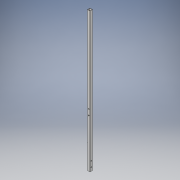
# Autodesk Inventor part: suporte sensores 1m
Saved by Autodesk Inventor 2019.4 (Build 234330000, 330)
## iProperties
Created: 2020-08-25
Part Number: suporte sensores 1m
Material: Alumínio 6061
Document SubType Name: Modeling
Designer: Lattes
Density: 2.7 g/cm^3
Appearance: Alumínio - Polido
Author: Lattes
Autodesk Inventor part; units mm, degrees
ref_plane "YZ Plane" through (0, 0, 0) normal (1, 0, 0) x (0, 1, 0)
ref_plane "XZ Plane" through (0, 0, 0) normal (0, 1, 0) x (-1, 0, 0)
ref_plane "XY Plane" through (0, 0, 0) normal (0, 0, 1) x (1, 0, 0)
sketch "Esboço1" plane through (0, 0, 0) normal (0, 1, 0) x (-1, 0, 0)
  line L0 (0, 0) -> (19.05, 0)
  line L1 (19.05, 0) -> (19.05, -19.05)
  line L2 (19.05, -19.05) -> (0, -19.05)
  line L3 (0, -19.05) -> (0, 0)
  line L4 (17.55, -17.55) -> (17.55, -1.5)
  line L5 (1.5, -1.5) -> (17.55, -1.5)
  line L6 (17.55, -17.55) -> (1.5, -17.55)
  line L7 (1.5, -1.5) -> (1.5, -17.55)
  dimension "d1" = 19.05
  dimension "d2" = 19.05
  dimension "d3" = 19.05
  constraints: 16 end point, 2 perpendicular, 1 horizontal
  measures "d1" distance of L0.start L0.end
  measures "d2" distance of L0.end L1.end
  measures "d3" distance of L1.end L2.end
extrude "Extrusão1" add sketch "Esboço1" along normal blind 1000
sketch "Esboço2" plane through (-19.05, 0, -19.05) normal (0, 0, -1) x (-1, 0, 0)
  point P0 (-19.05, 0)
sketch "Esboço3" plane through (0, 0, 0) normal (0, 0, 1) x (1, 0, 0)
  line L0 (-19.05, 0) -> (0, 0) projected
  line L1 (0, 0) -> (-19.05, 0)
  line L2 (-9.525, 0) -> (-9.525, 480)
  circle A0 centre (-9.525, 479.5) radius 3.5
  circle A1 centre (-9.525, 520.5) radius 3.5
  dimension "d15" = 480
  dimension "d56" = 7
  dimension "d57" = 7
  constraints: 4 end point, 2 centre point, 1 collinear, 1 midpoint, 1 vertical
  measures "d15" distance of L2.start L2.end
  measures "d56" diameter of A0
  measures "d57" diameter of A1
extrude "Extrusão2" cut sketch "Esboço3" against normal blind 20
sketch "Esboço6" plane through (0, 1000, 0) normal (0, 1, 0) x (1, 0, 0)
  line L0 (-19.05, 19.05) -> (0, 19.05) projected
  line L1 (0, 0) -> (-19.05, 0) projected
  line L2 (0, 19.05) -> (-19.05, 19.05)
  line L3 (-19.05, 19.05) -> (-19.05, 0)
  line L4 (-19.05, 0) -> (0, 0)
  line L5 (0, 0) -> (0, 19.05)
  line L6 (-17.55, 1.5) -> (-1.5, 1.5) projected
  line L7 (-17.55, 1.5) -> (-1.5, 1.5)
  line L8 (-1.5, 1.5) -> (-1.5, 17.55)
  line L9 (-1.5, 17.55) -> (-17.55, 17.55)
  line L10 (-17.55, 17.55) -> (-17.55, 1.5)
  constraints: 16 end point, 4 parallel, 2 horizontal, 2 perpendicular
extrude "Extrusão5" add sketch "Esboço6" along normal blind 150
chamfer "Chanfro1" distance 0.5 angle 45 4 edges at (0, 575, 0) (-17.55, 575, -1.5) (-19.05, 575, -19.05) (0, 575, -19.05)
chamfer "Chanfro2" distance 0.5 angle 45 1 edges at (-19.05, 575, 0)
sketch "Esboço7" plane through (-0.5, 0, 0) normal (0, 0, 1) x (1, 0, 0)
  point P0 (0.5, 0)
sketch "Esboço8" plane through (-19.05, 0, -18.55) normal (-1, 0, 0) x (0, 0, 1)
  line L0 (18.55, 1150) -> (16.55, 550.0033)
  line L1 (16.55, 0) -> (16.55, 1150) projected
  line L2 (16.55, 550.0033) -> (16.55, 150.0033)
  line L3 (16.55, 150.0033) -> (1, 150.0033)
  line L4 (1, 0) -> (1, 1150) projected
  line L5 (8.775, 150.0033) -> (8.775, 190.0033)
  circle A0 centre (8.775, 190.0033) radius 3.5
  circle A1 centre (8.775, 150.0033) radius 3.5
  point P0 (18.55, 0)
  dimension "d44" = 600
  dimension "d45" = 400
  dimension "d46" = 40
  dimension "d47" = 7
  dimension "d48" = 7
  constraints: 8 end point, 3 point on line, 2 centre point, 2 coincident, 1 horizontal, 1 midpoint, 1 vertical
  measures "d44" distance of L0.start L0.end
  measures "d45" distance of L0.end L2.end
  measures "d46" distance of L5.start L5.end
  measures "d47" diameter of A0
  measures "d48" diameter of A1
extrude "Extrusão6" cut sketch "Esboço8" against normal blind 100
sketch "Esboço9" plane through (-19.05, 0, -18.55) normal (-1, 0, 0) x (0, 0, 1)
  circle A0 centre (8.775, 150.0033) radius 3.5 projected
  line L0 (8.775, 150.0033) -> (8.775, 124.0033)
  line L1 (8.775, 124.0033) -> (55.0981, 124.0033)
  line L2 (18.55, 0) -> (-66.7734, 0)
  line L3 (55.0981, 124.0033) -> (-62.8208, 124.0033)
  line L4 (-62.8208, 124.0033) -> (-62.8208, 0)
  line L5 (-62.8208, 0) -> (55.0981, 0)
  line L6 (55.0981, 0) -> (55.0981, 124.0033)
  dimension "d51" = 26
  constraints: 14 end point, 2 horizontal, 2 parallel, 2 perpendicular, 1 point on line, 1 vertical
  measures "d51" distance of L0.start L0.end
extrude "Extrusão7" cut sketch "Esboço9" against normal blind 100 contours L1 L6 L5 L2 L4 L3
